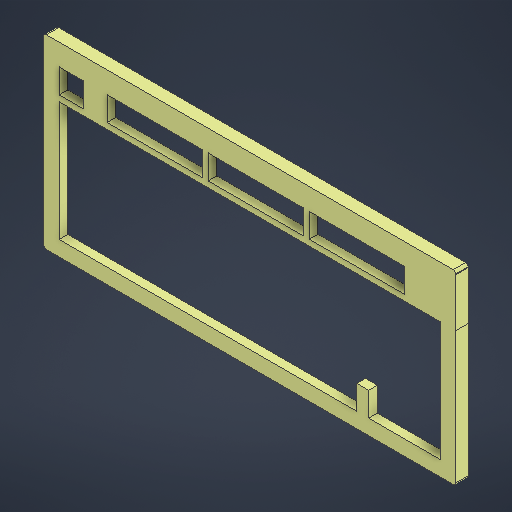
# Autodesk Inventor part: Keyboard_Case
Saved by Autodesk Inventor 2026.1 (Build 301233000, 233)
## iProperties
Created: 2025-11-09
Part Number: Keyboard_Case
Material: Generic
Document SubType Name: Modeling
Designer: avani
Density: 1 g/cm^3
Appearance: Default
Autodesk Inventor part; units mm, degrees
(part 1 of 5)
ref_plane "YZ Plane" through (0, 0, 0) normal (1, 0, 0) x (0, 1, 0)
ref_plane "XZ Plane" through (0, 0, 0) normal (0, 1, 0) x (-1, 0, 0)
sketch "Sketch1" plane through (0, 0, 0) normal (0, 0, 1) x (1, 0, 0)
  point P0 (0, 0)
sketch3d "3D 0"
sketch "Sketch2" plane through (0, 0, 0) normal (0, 0, 1) x (1, 0, 0)
  line L0 (303.652, 119.844) -> (303.808, 119.826) projected
  line L1 (303.808, 119.826) -> (303.962, 119.796) projected
  line L2 (303.962, 119.796) -> (304.115, 119.753) projected
  line L3 (304.115, 119.753) -> (304.261, 119.698) projected
  line L4 (304.261, 119.698) -> (304.403, 119.633) projected
  line L5 (304.403, 119.633) -> (304.541, 119.556) projected
  line L6 (304.672, 119.469) -> (304.794, 119.371) projected
  line L7 (304.541, 119.556) -> (304.672, 119.469) projected
  line L8 (304.794, 119.371) -> (304.91, 119.265) projected
  line L9 (304.91, 119.265) -> (305.016, 119.149) projected
  line L10 (305.016, 119.149) -> (305.114, 119.025) projected
  line L11 (305.114, 119.025) -> (305.201, 118.894) projected
  line L12 (305.201, 118.894) -> (305.278, 118.758) projected
  line L13 (305.278, 118.758) -> (305.343, 118.616) projected
  line L14 (305.343, 118.616) -> (305.398, 118.468) projected
  line L15 (305.398, 118.468) -> (305.441, 118.317) projected
  line L16 (305.441, 118.317) -> (305.471, 118.163) projected
  line L17 (305.471, 1.8741) -> (305.441, 1.7198) projected
  line L18 (305.398, 1.5696) -> (305.343, 1.4221) projected
  line L19 (305.343, 1.4221) -> (305.278, 1.2788) projected
  line L20 (305.278, 1.2788) -> (305.201, 1.1424) projected
  line L21 (305.201, 1.1424) -> (305.114, 1.0115) projected
  line L22 (305.441, 1.7198) -> (305.398, 1.5696) projected
  line L23 (305.114, 1.0115) -> (305.016, 0.8875) projected
  line L24 (305.016, 0.8875) -> (304.91, 0.7731) projected
  line L25 (304.794, 0.6656) -> (304.672, 0.5691) projected
  line L26 (304.672, 0.5691) -> (304.541, 0.4823) projected
  line L27 (304.541, 0.4823) -> (304.403, 0.4051) projected
  line L28 (304.91, 0.7731) -> (304.794, 0.6656) projected
  line L29 (304.403, 0.4051) -> (304.261, 0.339) projected
  line L30 (304.261, 0.339) -> (304.115, 0.2853) projected
  line L31 (304.115, 0.2853) -> (303.962, 0.2425) projected
  line L32 (303.962, 0.2425) -> (303.808, 0.2122) projected
  line L33 (303.808, 0.2122) -> (303.652, 0.1929) projected
  line L34 (303.652, 0.1929) -> (303.496, 0.1874) projected
  line L35 (305.471, 118.163) -> (305.489, 118.007) projected
  line L36 (305.489, 118.007) -> (305.496, 117.85) projected
  line L37 (305.496, 117.85) -> (305.496, 2.1869) projected
  line L38 (305.496, 2.1869) -> (305.489, 2.0299) projected
  line L39 (305.489, 2.0299) -> (305.471, 1.8741) projected
  line L40 (2.096, 119.849) -> (303.496, 119.849) projected
  line L41 (303.496, 0.1874) -> (2.096, 0.1874) projected
  line L42 (135.883, 116.926) -> (135.883, 103.125) projected
  line L43 (135.883, 103.125) -> (122.083, 103.125) projected
  line L44 (122.083, 116.926) -> (135.883, 116.926) projected
  line L45 (122.083, 103.125) -> (122.083, 116.926) projected
  line L46 (98.2694, 116.926) -> (112.07, 116.926) projected
  line L47 (112.07, 103.125) -> (98.2694, 103.125) projected
  line L48 (112.07, 116.926) -> (112.07, 103.125) projected
  line L49 (28.7266, 35.9625) -> (14.9269, 35.9625) projected
  line L50 (23.9641, 55.0125) -> (23.9641, 41.2129) projected
  line L51 (23.9641, 41.2129) -> (10.163, 41.2129) projected
  line L52 (10.163, 55.0125) -> (23.9641, 55.0125) projected
  line L53 (10.163, 41.2129) -> (10.163, 55.0125) projected
  line L54 (78.0881, 15.4423) -> (78.0881, 12.2136) projected
  line L55 (78.0881, 12.2136) -> (77.264, 12.2136) projected
  line L56 (77.264, 12.2136) -> (77.264, 9.6132) projected
  line L57 (77.264, 9.6132) -> (78.0881, 9.6132) projected
  line L58 (53.0271, 16.9127) -> (66.8267, 16.9127) projected
  line L59 (66.8267, 16.9127) -> (66.8267, 3.113) projected
  line L60 (53.0271, 3.113) -> (53.0271, 16.9127) projected
  line L61 (66.8267, 3.113) -> (53.0271, 3.113) projected
  line L62 (78.0881, 9.6132) -> (78.0881, 3.3431) projected
  line L63 (78.7329, 22.163) -> (64.9333, 22.163) projected
  line L64 (78.7329, 35.9625) -> (78.7329, 22.163) projected
  line L65 (64.9333, 35.9625) -> (78.7329, 35.9625) projected
  line L66 (69.2079, 41.2129) -> (55.4083, 41.2129) projected
  line L67 (69.2079, 55.0125) -> (69.2079, 41.2129) projected
  line L68 (55.4083, 55.0125) -> (69.2079, 55.0125) projected
  line L69 (55.4083, 41.2129) -> (55.4083, 55.0125) projected
  line L70 (50.1579, 55.0125) -> (50.1579, 41.2129) projected
  line L71 (50.1579, 41.2129) -> (36.3583, 41.2129) projected
  line L72 (36.3583, 55.0125) -> (50.1579, 55.0125) projected
  line L73 (36.3583, 41.2129) -> (36.3583, 55.0125) projected
  line L74 (84.6391, 15.4423) -> (78.0881, 15.4423) projected
  line L75 (78.0881, 3.3431) -> (79.8132, 3.3431) projected
  line L76 (84.6391, 3.3431) -> (84.6391, 7.8135) projected
  line L77 (82.9137, 3.3431) -> (84.6391, 3.3431) projected
  line L78 (82.9137, 2.1429) -> (82.9137, 3.3431) projected
  line L79 (79.8132, 2.1429) -> (82.9137, 2.1429) projected
  line L80 (79.8132, 3.3431) -> (79.8132, 2.1429) projected
  line L81 (21.5828, 60.2629) -> (7.7832, 60.2629) projected
  line L82 (7.7832, 74.0625) -> (21.5828, 74.0625) projected
  line L83 (7.7832, 60.2629) -> (7.7832, 74.0625) projected
  line L84 (21.5828, 74.0625) -> (21.5828, 60.2629) projected
  line L85 (31.5957, 60.2629) -> (31.5957, 74.0625) projected
  line L86 (35.8704, 79.3129) -> (22.0707, 79.3129) projected
  line L87 (45.3954, 60.2629) -> (31.5957, 60.2629) projected
  line L88 (31.5957, 74.0625) -> (45.3954, 74.0625) projected
  line L89 (45.3954, 74.0625) -> (45.3954, 60.2629) projected
  line L90 (0.0951, 2.1869) -> (0.0951, 117.85) projected
  line L91 (16.8203, 79.3129) -> (3.0193, 79.3129) projected
  line L92 (3.0193, 79.3129) -> (3.0193, 93.1125) projected
  line L93 (16.8203, 93.1125) -> (16.8203, 79.3129) projected
  line L94 (3.0193, 93.1125) -> (16.8203, 93.1125) projected
  line L95 (16.8203, 103.125) -> (3.0193, 103.125) projected
  line L96 (3.0193, 103.125) -> (3.0193, 116.926) projected
  line L97 (3.0193, 116.926) -> (16.8203, 116.926) projected
  line L98 (16.8203, 116.926) -> (16.8203, 103.125) projected
  line L99 (124.463, 12.2136) -> (84.6391, 12.2136) projected
  line L100 (84.6391, 12.2136) -> (84.6391, 15.4423) projected
  line L101 (84.6391, 7.8135) -> (124.463, 7.8135) projected
  line L102 (97.7829, 35.9625) -> (97.7829, 22.163) projected
  line L103 (103.033, 22.163) -> (103.033, 35.9625) projected
  line L104 (116.833, 22.163) -> (103.033, 22.163) projected
  line L105 (116.833, 35.9625) -> (116.833, 22.163) projected
  line L106 (103.033, 35.9625) -> (116.833, 35.9625) projected
  line L107 (97.7829, 22.163) -> (83.9833, 22.163) projected
  line L108 (83.9833, 22.163) -> (83.9833, 35.9625) projected
  line L109 (107.308, 41.2129) -> (93.5083, 41.2129) projected
  line L110 (83.9833, 35.9625) -> (97.7829, 35.9625) projected
  line L111 (93.5083, 55.0125) -> (107.308, 55.0125) projected
  line L112 (93.5083, 41.2129) -> (93.5083, 55.0125) projected
  line L113 (22.0707, 93.1125) -> (35.8704, 93.1125) projected
  line L114 (22.0707, 79.3129) -> (22.0707, 93.1125) projected
  line L115 (35.8704, 93.1125) -> (35.8704, 79.3129) projected
  line L116 (41.1208, 79.3129) -> (41.1208, 93.1125) projected
  line L117 (54.919, 79.3129) -> (41.1208, 79.3129) projected
  line L118 (54.919, 93.1125) -> (54.919, 79.3129) projected
  line L119 (74.4583, 41.2129) -> (74.4583, 55.0125) projected
  line L120 (83.4954, 60.2629) -> (69.6958, 60.2629) projected
  line L121 (69.6958, 60.2629) -> (69.6958, 74.0625) projected
  line L122 (83.4954, 74.0625) -> (83.4954, 60.2629) projected
  line L123 (74.4583, 55.0125) -> (88.2579, 55.0125) projected
  line L124 (88.2579, 55.0125) -> (88.2579, 41.2129) projected
  line L125 (88.2579, 41.2129) -> (74.4583, 41.2129) projected
  line L126 (50.6458, 74.0625) -> (64.4454, 74.0625) projected
  line L127 (64.4454, 74.0625) -> (64.4454, 60.2629) projected
  line L128 (64.4454, 60.2629) -> (50.6458, 60.2629) projected
  line L129 (50.6458, 60.2629) -> (50.6458, 74.0625) projected
  line L130 (73.9704, 79.3129) -> (60.1694, 79.3129) projected
  line L131 (79.2194, 79.3129) -> (79.2194, 93.1125) projected
  line L132 (73.9704, 93.1125) -> (73.9704, 79.3129) projected
  line L133 (60.1694, 93.1125) -> (73.9704, 93.1125) projected
  line L134 (60.1694, 79.3129) -> (60.1694, 93.1125) projected
  line L135 (69.6958, 74.0625) -> (83.4954, 74.0625) projected
  line L136 (107.794, 60.2629) -> (107.794, 74.0625) projected
  line L137 (102.545, 74.0625) -> (102.545, 60.2629) projected
  line L138 (102.545, 60.2629) -> (88.7444, 60.2629) projected
  line L139 (88.7444, 74.0625) -> (102.545, 74.0625) projected
  line L140 (88.7444, 60.2629) -> (88.7444, 74.0625) projected
  line L141 (54.919, 103.125) -> (41.1208, 103.125) projected
  line L142 (54.919, 116.926) -> (54.919, 103.125) projected
  line L143 (41.1208, 103.125) -> (41.1208, 116.926) projected
  line L144 (41.1208, 116.926) -> (54.919, 116.926) projected
  line L145 (41.1208, 93.1125) -> (54.919, 93.1125) projected
  line L146 (0.0951, 117.85) -> (0.102, 118.007) projected
  line L147 (0.102, 118.007) -> (0.1199, 118.163) projected
  line L148 (0.1199, 118.163) -> (0.1502, 118.317) projected
  line L149 (0.4768, 119.025) -> (0.5746, 119.149) projected
  line L150 (0.39, 118.894) -> (0.4768, 119.025) projected
  line L151 (0.3128, 118.758) -> (0.39, 118.894) projected
  line L152 (0.248, 118.616) -> (0.3128, 118.758) projected
  line L153 (0.1929, 118.468) -> (0.248, 118.616) projected
  line L154 (0.1502, 118.317) -> (0.1929, 118.468) projected
  line L155 (0.5746, 119.149) -> (0.6808, 119.265) projected
  line L156 (0.6808, 119.265) -> (0.7965, 119.371) projected
  line L157 (0.7965, 119.371) -> (0.9192, 119.469) projected
  line L158 (0.9192, 119.469) -> (1.0501, 119.556) projected
  line L159 (1.0501, 119.556) -> (1.1879, 119.633) projected
  line L160 (1.1879, 119.633) -> (1.3298, 119.698) projected
  line L161 (1.3298, 119.698) -> (1.4759, 119.753) projected
  line L162 (1.4759, 119.753) -> (1.6288, 119.796) projected
  line L163 (1.6288, 119.796) -> (1.7818, 119.826) projected
  line L164 (1.7818, 119.826) -> (1.9389, 119.844) projected
  line L165 (1.9389, 119.844) -> (2.096, 119.849) projected
  line L166 (107.308, 55.0125) -> (107.308, 41.2129) projected
  line L167 (112.558, 41.2129) -> (112.558, 55.0125) projected
  line L168 (126.358, 41.2129) -> (112.558, 41.2129) projected
  line L169 (126.358, 55.0125) -> (126.358, 41.2129) projected
  line L170 (112.558, 55.0125) -> (126.358, 55.0125) projected
  line L171 (121.595, 60.2629) -> (107.794, 60.2629) projected
  line L172 (107.794, 74.0625) -> (121.595, 74.0625) projected
  line L173 (121.595, 74.0625) -> (121.595, 60.2629) projected
  line L174 (93.0204, 79.3129) -> (79.2194, 79.3129) projected
  line L175 (93.0204, 93.1125) -> (93.0204, 79.3129) projected
  line L176 (79.2194, 93.1125) -> (93.0204, 93.1125) projected
  line L177 (93.0204, 103.125) -> (79.2194, 103.125) projected
  line L178 (98.2694, 103.125) -> (98.2694, 116.926) projected
  line L179 (145.896, 74.0625) -> (159.695, 74.0625) projected
  line L180 (159.695, 74.0625) -> (159.695, 60.2629) projected
  line L181 (145.896, 60.2629) -> (145.896, 74.0625) projected
  line L182 (140.645, 74.0625) -> (140.645, 60.2629) projected
  line L183 (140.645, 60.2629) -> (126.846, 60.2629) projected
  line L184 (126.846, 74.0625) -> (140.645, 74.0625) projected
  line L185 (126.846, 60.2629) -> (126.846, 74.0625) projected
  line L186 (112.07, 79.3129) -> (98.2694, 79.3129) projected
  line L187 (98.2694, 93.1125) -> (112.07, 93.1125) projected
  line L188 (98.2694, 79.3129) -> (98.2694, 93.1125) projected
  line L189 (131.12, 79.3129) -> (117.321, 79.3129) projected
  line L190 (112.07, 93.1125) -> (112.07, 79.3129) projected
  line L191 (117.321, 79.3129) -> (117.321, 93.1125) projected
  line L192 (131.12, 93.1125) -> (131.12, 79.3129) projected
  line L193 (117.321, 93.1125) -> (131.12, 93.1125) projected
  line L194 (79.2194, 116.926) -> (93.0204, 116.926) projected
  line L195 (93.0204, 116.926) -> (93.0204, 103.125) projected
  line L196 (79.2194, 103.125) -> (79.2194, 116.926) projected
  line L197 (73.9704, 103.125) -> (60.1694, 103.125) projected
  line L198 (73.9704, 116.926) -> (73.9704, 103.125) projected
  line L199 (60.1694, 103.125) -> (60.1694, 116.926) projected
  line L200 (60.1694, 116.926) -> (73.9704, 116.926) projected
  line L201 (141.133, 22.163) -> (141.133, 35.9625) projected
  line L202 (141.133, 35.9625) -> (154.933, 35.9625) projected
  line L203 (138.264, 7.8135) -> (178.088, 7.8135) projected
  line L204 (178.088, 12.2136) -> (138.264, 12.2136) projected
  line L205 (154.933, 35.9625) -> (154.933, 22.163) projected
  line L206 (178.088, 15.4423) -> (178.088, 12.2136) projected
  line L207 (160.183, 22.163) -> (160.183, 35.9625) projected
  line L208 (173.983, 22.163) -> (160.183, 22.163) projected
  line L209 (160.183, 35.9625) -> (173.983, 35.9625) projected
  line L210 (173.983, 35.9625) -> (173.983, 22.163) projected
  line L211 (184.638, 12.2136) -> (184.638, 15.4423) projected
  line L212 (184.638, 15.4423) -> (178.088, 15.4423) projected
  line L213 (193.033, 22.163) -> (179.233, 22.163) projected
  line L214 (179.233, 22.163) -> (179.233, 35.9625) projected
  line L215 (179.233, 35.9625) -> (193.033, 35.9625) projected
  line L216 (193.033, 35.9625) -> (193.033, 22.163) projected
  line L217 (178.088, 7.8135) -> (178.088, 3.3431) projected
  line L218 (178.088, 3.3431) -> (179.813, 3.3431) projected
  line L219 (179.813, 3.3431) -> (179.813, 2.1429) projected
  line L220 (179.813, 2.1429) -> (182.914, 2.1429) projected
  line L221 (182.914, 2.1429) -> (182.914, 3.3431) projected
  line L222 (185.463, 12.2136) -> (184.638, 12.2136) projected
  line L223 (185.463, 9.6132) -> (185.463, 12.2136) projected
  line L224 (184.638, 9.6132) -> (185.463, 9.6132) projected
  line L225 (184.638, 3.3431) -> (184.638, 9.6132) projected
  line L226 (182.914, 3.3431) -> (184.638, 3.3431) projected
  line L227 (195.902, 16.9127) -> (209.702, 16.9127) projected
  line L228 (209.702, 16.9127) -> (209.702, 3.113) projected
  line L229 (209.702, 3.113) -> (195.902, 3.113) projected
  line L230 (195.902, 3.113) -> (195.902, 16.9127) projected
  line L231 (124.463, 16.9127) -> (124.463, 12.2136) projected
  line L232 (124.463, 7.8135) -> (124.463, 3.113) projected
  line L233 (124.463, 3.113) -> (138.264, 3.113) projected
  line L234 (138.264, 12.2136) -> (138.264, 16.9127) projected
  line L235 (138.264, 16.9127) -> (124.463, 16.9127) projected
  line L236 (122.083, 35.9625) -> (135.883, 35.9625) projected
  line L237 (135.883, 22.163) -> (122.083, 22.163) projected
  line L238 (122.083, 22.163) -> (122.083, 35.9625) projected
  line L239 (135.883, 35.9625) -> (135.883, 22.163) projected
  line L240 (138.264, 3.113) -> (138.264, 7.8135) projected
  line L241 (154.933, 22.163) -> (141.133, 22.163) projected
  line L242 (202.558, 41.2129) -> (188.758, 41.2129) projected
  line L243 (188.758, 41.2129) -> (188.758, 55.0125) projected
  line L244 (188.758, 55.0125) -> (202.558, 55.0125) projected
  line L245 (202.558, 55.0125) -> (202.558, 41.2129) projected
  line L246 (221.608, 55.0125) -> (221.608, 41.2129) projected
  line L247 (226.858, 41.2129) -> (226.858, 55.0125) projected
  line L248 (240.658, 41.2129) -> (226.858, 41.2129) projected
  line L249 (240.658, 55.0125) -> (240.658, 41.2129) projected
  line L250 (257.813, 55.0125) -> (257.813, 50.3135) projected
  line L251 (257.813, 50.3135) -> (256.089, 50.3135) projected
  line L252 (256.089, 50.3135) -> (256.089, 53.5421) projected
  line L253 (256.089, 53.5421) -> (249.538, 53.5421) projected
  line L254 (248.714, 47.7132) -> (249.538, 47.7132) projected
  line L255 (249.538, 50.3135) -> (248.714, 50.3135) projected
  line L256 (248.714, 50.3135) -> (248.714, 47.7132) projected
  line L257 (249.538, 53.5421) -> (249.538, 50.3135) projected
  line L258 (257.813, 45.9133) -> (257.813, 41.2129) projected
  line L259 (256.089, 45.9133) -> (257.813, 45.9133) projected
  line L260 (257.813, 41.2129) -> (271.614, 41.2129) projected
  line L261 (256.089, 41.4433) -> (256.089, 45.9133) projected
  line L262 (271.614, 45.9133) -> (273.338, 45.9133) projected
  line L263 (273.338, 45.9133) -> (273.338, 41.4433) projected
  line L264 (273.338, 41.4433) -> (275.063, 41.4433) projected
  line L265 (271.614, 41.2129) -> (271.614, 45.9133) projected
  line L266 (273.338, 50.3135) -> (271.614, 50.3135) projected
  line L267 (271.614, 50.3135) -> (271.614, 55.0125) projected
  line L268 (273.338, 53.5421) -> (273.338, 50.3135) projected
  line L269 (278.758, 60.2629) -> (264.958, 60.2629) projected
  line L270 (271.614, 55.0125) -> (257.813, 55.0125) projected
  line L271 (278.758, 74.0625) -> (278.758, 60.2629) projected
  line L272 (264.958, 74.0625) -> (278.758, 74.0625) projected
  line L273 (264.958, 60.2629) -> (264.958, 74.0625) projected
  line L274 (260.196, 79.3129) -> (273.995, 79.3129) projected
  line L275 (150.17, 79.3129) -> (136.371, 79.3129) projected
  line L276 (169.22, 79.3129) -> (155.421, 79.3129) projected
  line L277 (136.371, 93.1125) -> (150.17, 93.1125) projected
  line L278 (136.371, 79.3129) -> (136.371, 93.1125) projected
  line L279 (150.17, 93.1125) -> (150.17, 79.3129) projected
  line L280 (155.421, 79.3129) -> (155.421, 93.1125) projected
  line L281 (169.22, 93.1125) -> (169.22, 79.3129) projected
  line L282 (155.421, 93.1125) -> (169.22, 93.1125) projected
  line L283 (173.983, 103.125) -> (160.183, 103.125) projected
  line L284 (154.933, 103.125) -> (141.133, 103.125) projected
  line L285 (141.133, 103.125) -> (141.133, 116.926) projected
  line L286 (141.133, 116.926) -> (154.933, 116.926) projected
  line L287 (154.933, 116.926) -> (154.933, 103.125) projected
  line L288 (160.183, 103.125) -> (160.183, 116.926) projected
  line L289 (160.183, 116.926) -> (173.983, 116.926) projected
  line L290 (173.983, 116.926) -> (173.983, 103.125) projected
  line L291 (178.745, 74.0625) -> (178.745, 60.2629) projected
  line L292 (178.745, 60.2629) -> (164.946, 60.2629) projected
  line L293 (164.946, 60.2629) -> (164.946, 74.0625) projected
  line L294 (164.946, 74.0625) -> (178.745, 74.0625) projected
  line L295 (197.795, 60.2629) -> (183.996, 60.2629) projected
  line L296 (197.795, 74.0625) -> (197.795, 60.2629) projected
  line L297 (183.996, 60.2629) -> (183.996, 74.0625) projected
  line L298 (183.996, 74.0625) -> (197.795, 74.0625) projected
  line L299 (183.508, 55.0125) -> (183.508, 41.2129) projected
  line L300 (183.508, 41.2129) -> (169.708, 41.2129) projected
  line L301 (169.708, 41.2129) -> (169.708, 55.0125) projected
  line L302 (169.708, 55.0125) -> (183.508, 55.0125) projected
  line L303 (188.27, 79.3129) -> (174.471, 79.3129) projected
  line L304 (207.32, 79.3129) -> (193.521, 79.3129) projected
  line L305 (174.471, 93.1125) -> (188.27, 93.1125) projected
  line L306 (174.471, 79.3129) -> (174.471, 93.1125) projected
  line L307 (188.27, 93.1125) -> (188.27, 79.3129) projected
  line L308 (193.521, 79.3129) -> (193.521, 93.1125) projected
  line L309 (207.32, 93.1125) -> (207.32, 79.3129) projected
  line L310 (193.521, 93.1125) -> (207.32, 93.1125) projected
  line L311 (216.845, 74.0625) -> (216.845, 60.2629) projected
  line L312 (216.845, 60.2629) -> (203.046, 60.2629) projected
  line L313 (203.046, 60.2629) -> (203.046, 74.0625) projected
  line L314 (203.046, 74.0625) -> (216.845, 74.0625) projected
  line L315 (216.845, 103.125) -> (203.046, 103.125) projected
  line L316 (193.033, 103.125) -> (179.233, 103.125) projected
  line L317 (179.233, 103.125) -> (179.233, 116.926) projected
  line L318 (179.233, 116.926) -> (193.033, 116.926) projected
  line L319 (193.033, 116.926) -> (193.033, 103.125) projected
  line L320 (203.046, 103.125) -> (203.046, 116.926) projected
  line L321 (216.845, 116.926) -> (216.845, 103.125) projected
  line L322 (203.046, 116.926) -> (216.845, 116.926) projected
  line L323 (235.895, 60.2629) -> (222.096, 60.2629) projected
  line L324 (222.096, 60.2629) -> (222.096, 74.0625) projected
  line L325 (222.096, 74.0625) -> (235.895, 74.0625) projected
  line L326 (235.895, 74.0625) -> (235.895, 60.2629) projected
  line L327 (226.858, 55.0125) -> (240.658, 55.0125) projected
  line L328 (198.283, 35.9625) -> (212.083, 35.9625) projected
  line L329 (212.083, 35.9625) -> (212.083, 22.163) projected
  line L330 (212.083, 22.163) -> (198.283, 22.163) projected
  line L331 (207.808, 55.0125) -> (221.608, 55.0125) projected
  line L332 (207.808, 41.2129) -> (207.808, 55.0125) projected
  line L333 (217.333, 35.9625) -> (231.133, 35.9625) projected
  line L334 (231.133, 35.9625) -> (231.133, 22.163) projected
  line L335 (231.133, 22.163) -> (217.333, 22.163) projected
  line L336 (221.608, 41.2129) -> (207.808, 41.2129) projected
  line L337 (198.283, 22.163) -> (198.283, 35.9625) projected
  line L338 (217.333, 22.163) -> (217.333, 35.9625) projected
  line L339 (226.37, 79.3129) -> (212.571, 79.3129) projected
  line L340 (245.42, 79.3129) -> (231.621, 79.3129) projected
  line L341 (212.571, 93.1125) -> (226.37, 93.1125) projected
  line L342 (212.571, 79.3129) -> (212.571, 93.1125) projected
  line L343 (226.37, 93.1125) -> (226.37, 79.3129) projected
  line L344 (231.621, 79.3129) -> (231.621, 93.1125) projected
  line L345 (245.42, 93.1125) -> (245.42, 79.3129) projected
  line L346 (231.621, 93.1125) -> (245.42, 93.1125) projected
  line L347 (235.895, 103.125) -> (222.096, 103.125) projected
  line L348 (254.945, 103.125) -> (241.146, 103.125) projected
  line L349 (241.146, 116.926) -> (254.945, 116.926) projected
  line L350 (241.146, 103.125) -> (241.146, 116.926) projected
  line L351 (222.096, 103.125) -> (222.096, 116.926) projected
  line L352 (222.096, 116.926) -> (235.895, 116.926) projected
  line L353 (235.895, 116.926) -> (235.895, 103.125) projected
  line L354 (241.146, 74.0625) -> (254.945, 74.0625) projected
  line L355 (254.945, 74.0625) -> (254.945, 60.2629) projected
  line L356 (254.945, 60.2629) -> (241.146, 60.2629) projected
  line L357 (241.146, 60.2629) -> (241.146, 74.0625) projected
  line L358 (251.92, 85.8132) -> (251.92, 79.5433) projected
  line L359 (251.92, 79.5433) -> (253.646, 79.5433) projected
  line L360 (256.745, 78.3428) -> (256.745, 79.5433) projected
  line L361 (253.646, 79.5433) -> (253.646, 78.3428) projected
  line L362 (253.646, 78.3428) -> (256.745, 78.3428) projected
  line L363 (256.745, 79.5433) -> (258.47, 79.5433) projected
  line L364 (260.196, 84.0133) -> (260.196, 79.3129) projected
  line L365 (258.47, 84.0133) -> (260.196, 84.0133) projected
  line L366 (258.47, 79.5433) -> (258.47, 84.0133) projected
  line L367 (260.196, 93.1125) -> (260.196, 88.4135) projected
  line L368 (260.196, 88.4135) -> (258.47, 88.4135) projected
  line L369 (251.095, 85.8132) -> (251.92, 85.8132) projected
  line L370 (251.095, 88.4135) -> (251.095, 85.8132) projected
  line L371 (251.92, 88.4135) -> (251.095, 88.4135) projected
  line L372 (251.92, 91.6421) -> (251.92, 88.4135) projected
  line L373 (258.47, 91.6421) -> (251.92, 91.6421) projected
  line L374 (258.47, 88.4135) -> (258.47, 91.6421) projected
  line L375 (273.995, 93.1125) -> (260.196, 93.1125) projected
  line L376 (273.995, 103.125) -> (260.196, 103.125) projected
  line L377 (273.995, 116.926) -> (273.995, 103.125) projected
  line L378 (260.196, 116.926) -> (273.995, 116.926) projected
  line L379 (260.196, 103.125) -> (260.196, 116.926) projected
  line L380 (254.945, 116.926) -> (254.945, 103.125) projected
  line L381 (249.538, 47.7132) -> (249.538, 41.4433) projected
  line L382 (249.538, 41.4433) -> (251.263, 41.4433) projected
  line L383 (251.263, 41.4433) -> (251.263, 40.2428) projected
  line L384 (251.263, 40.2428) -> (254.362, 40.2428) projected
  line L385 (254.362, 40.2428) -> (254.362, 41.4433) projected
  line L386 (254.362, 41.4433) -> (256.089, 41.4433) projected
  line L387 (164.458, 41.2129) -> (150.658, 41.2129) projected
  line L388 (164.458, 55.0125) -> (164.458, 41.2129) projected
  line L389 (150.658, 55.0125) -> (164.458, 55.0125) projected
  line L390 (150.658, 41.2129) -> (150.658, 55.0125) projected
  line L391 (159.695, 60.2629) -> (145.896, 60.2629) projected
  line L392 (145.408, 55.0125) -> (145.408, 41.2129) projected
  line L393 (145.408, 41.2129) -> (131.608, 41.2129) projected
  line L394 (131.608, 55.0125) -> (145.408, 55.0125) projected
  line L395 (131.608, 41.2129) -> (131.608, 55.0125) projected
  line L396 (0.7965, 0.6656) -> (0.6808, 0.7731) projected
  line L397 (0.6808, 0.7731) -> (0.5746, 0.8875) projected
  line L398 (0.5746, 0.8875) -> (0.4768, 1.0115) projected
  line L399 (0.4768, 1.0115) -> (0.39, 1.1424) projected
  line L400 (0.39, 1.1424) -> (0.3128, 1.2788) projected
  line L401 (0.3128, 1.2788) -> (0.248, 1.4221) projected
  line L402 (14.9269, 35.9625) -> (14.9269, 31.2636) projected
  line L403 (14.9269, 31.2636) -> (13.2016, 31.2636) projected
  line L404 (13.2016, 31.2636) -> (13.2016, 34.4923) projected
  line L405 (13.2016, 34.4923) -> (6.6518, 34.4923) projected
  line L406 (6.6518, 34.4923) -> (6.6518, 31.2636) projected
  line L407 (6.6518, 31.2636) -> (5.8263, 31.2636) projected
  line L408 (5.8263, 31.2636) -> (5.8263, 28.6632) projected
  line L409 (5.8263, 28.6632) -> (6.6518, 28.6632) projected
  line L410 (30.4519, 26.8635) -> (30.4519, 22.3931) projected
  line L411 (30.4519, 22.3931) -> (32.1758, 22.3931) projected
  line L412 (32.1758, 22.3931) -> (32.1758, 21.1928) projected
  line L413 (32.1758, 21.1928) -> (35.2764, 21.1928) projected
  line L414 (35.2764, 21.1928) -> (35.2764, 22.3931) projected
  line L415 (35.2764, 22.3931) -> (37.0018, 22.3931) projected
  line L416 (37.0018, 22.3931) -> (37.0018, 28.6632) projected
  line L417 (37.0018, 28.6632) -> (37.8273, 28.6632) projected
  line L418 (37.8273, 28.6632) -> (37.8273, 31.2636) projected
  line L419 (37.8273, 31.2636) -> (37.0018, 31.2636) projected
  line L420 (37.0018, 31.2636) -> (37.0018, 34.4923) projected
  line L421 (37.0018, 34.4923) -> (30.4519, 34.4923) projected
  line L422 (30.4519, 31.2636) -> (28.7266, 31.2636) projected
  line L423 (28.7266, 31.2636) -> (28.7266, 35.9625) projected
  line L424 (30.4519, 34.4923) -> (30.4519, 31.2636) projected
  line L425 (13.2016, 26.8635) -> (14.9269, 26.8635) projected
  line L426 (13.2016, 22.3931) -> (13.2016, 26.8635) projected
  line L427 (6.6518, 28.6632) -> (6.6518, 22.3931) projected
  line L428 (6.6518, 22.3931) -> (8.3771, 22.3931) projected
  line L429 (29.213, 16.9127) -> (43.0142, 16.9127) projected
  line L430 (43.0142, 16.9127) -> (43.0142, 3.113) projected
  line L431 (43.0142, 3.113) -> (29.213, 3.113) projected
  line L432 (29.213, 3.113) -> (29.213, 16.9127) projected
  line L433 (14.9269, 26.8635) -> (14.9269, 22.163) projected
  line L434 (14.9269, 22.163) -> (28.7266, 22.163) projected
  line L435 (28.7266, 22.163) -> (28.7266, 26.8635) projected
  line L436 (28.7266, 26.8635) -> (30.4519, 26.8635) projected
  line L437 (8.3771, 22.3931) -> (8.3771, 21.1928) projected
  line L438 (11.4763, 21.1928) -> (11.4763, 22.3931) projected
  line L439 (8.3771, 21.1928) -> (11.4763, 21.1928) projected
  line L440 (5.4019, 16.9127) -> (19.2016, 16.9127) projected
  line L441 (5.4019, 3.113) -> (5.4019, 16.9127) projected
  line L442 (19.2016, 3.113) -> (5.4019, 3.113) projected
  line L443 (19.2016, 16.9127) -> (19.2016, 3.113) projected
  line L444 (11.4763, 22.3931) -> (13.2016, 22.3931) projected
  line L445 (0.248, 1.4221) -> (0.1929, 1.5696) projected
  line L446 (0.1929, 1.5696) -> (0.1502, 1.7198) projected
  line L447 (0.1502, 1.7198) -> (0.1199, 1.8741) projected
  line L448 (0.1199, 1.8741) -> (0.102, 2.0299) projected
  line L449 (0.102, 2.0299) -> (0.0951, 2.1869) projected
  line L450 (2.096, 0.1874) -> (1.9389, 0.1929) projected
  line L451 (1.9389, 0.1929) -> (1.7818, 0.2122) projected
  line L452 (1.7818, 0.2122) -> (1.6288, 0.2425) projected
  line L453 (0.9192, 0.5691) -> (0.7965, 0.6656) projected
  line L454 (1.0501, 0.4823) -> (0.9192, 0.5691) projected
  line L455 (1.3298, 0.339) -> (1.1879, 0.4051) projected
  line L456 (1.4759, 0.2853) -> (1.3298, 0.339) projected
  line L457 (1.6288, 0.2425) -> (1.4759, 0.2853) projected
  line L458 (1.1879, 0.4051) -> (1.0501, 0.4823) projected
  line L459 (64.9333, 22.163) -> (64.9333, 35.9625) projected
  line L460 (59.6829, 35.9625) -> (59.6829, 22.163) projected
  line L461 (59.6829, 22.163) -> (45.8833, 22.163) projected
  line L462 (45.8833, 22.163) -> (45.8833, 35.9625) projected
  line L463 (45.8833, 35.9625) -> (59.6829, 35.9625) projected
  line L464 (288.771, 35.9625) -> (302.57, 35.9625) projected
  line L465 (302.57, 35.9625) -> (302.57, 22.163) projected
  line L466 (288.771, 22.163) -> (288.771, 35.9625) projected
  line L467 (283.52, 22.163) -> (269.721, 22.163) projected
  line L468 (269.721, 35.9625) -> (283.52, 35.9625) projected
  line L469 (269.721, 22.163) -> (269.721, 35.9625) projected
  line L470 (283.52, 35.9625) -> (283.52, 22.163) projected
  line L471 (269.721, 16.9127) -> (283.52, 16.9127) projected
  line L472 (283.52, 16.9127) -> (283.52, 3.113) projected
  line L473 (283.52, 3.113) -> (269.721, 3.113) projected
  line L474 (269.721, 3.113) -> (269.721, 16.9127) projected
  line L475 (302.57, 22.163) -> (288.771, 22.163) projected
  line L476 (288.771, 16.9127) -> (302.57, 16.9127) projected
  line L477 (288.771, 3.113) -> (288.771, 16.9127) projected
  line L478 (302.57, 16.9127) -> (302.57, 3.113) projected
  line L479 (302.57, 3.113) -> (288.771, 3.113) projected
  line L480 (302.57, 41.2129) -> (288.771, 41.2129) projected
  line L481 (279.888, 47.7132) -> (280.713, 47.7132) projected
  line L482 (280.713, 50.3135) -> (279.888, 50.3135) projected
  line L483 (280.713, 47.7132) -> (280.713, 50.3135) projected
  line L484 (279.888, 50.3135) -> (279.888, 53.5421) projected
  line L485 (288.771, 41.2129) -> (288.771, 55.0125) projected
  line L486 (302.57, 55.0125) -> (302.57, 41.2129) projected
  line L487 (219.713, 16.9127) -> (233.514, 16.9127) projected
  line L488 (233.514, 16.9127) -> (233.514, 3.113) projected
  line L489 (233.514, 3.113) -> (219.713, 3.113) projected
  line L490 (219.713, 3.113) -> (219.713, 16.9127) projected
  line L491 (250.671, 16.9127) -> (264.47, 16.9127) projected
  line L492 (264.47, 16.9127) -> (264.47, 3.113) projected
  line L493 (264.47, 3.113) -> (250.671, 3.113) projected
  line L494 (250.671, 3.113) -> (250.671, 16.9127) projected
  line L495 (288.771, 55.0125) -> (302.57, 55.0125) projected
  line L496 (302.57, 60.2629) -> (288.771, 60.2629) projected
  line L497 (288.771, 60.2629) -> (288.771, 74.0625) projected
  line L498 (302.57, 74.0625) -> (302.57, 60.2629) projected
  line L499 (288.771, 74.0625) -> (302.57, 74.0625) projected
  line L500 (277.446, 78.3428) -> (280.545, 78.3428) projected
  line L501 (277.446, 79.5433) -> (277.446, 78.3428) projected
  line L502 (275.721, 79.5433) -> (277.446, 79.5433) projected
  line L503 (273.995, 79.3129) -> (273.995, 84.0133) projected
  line L504 (273.995, 84.0133) -> (275.721, 84.0133) projected
  line L505 (275.721, 84.0133) -> (275.721, 79.5433) projected
  line L506 (282.271, 88.4135) -> (282.271, 91.6421) projected
  line L507 (275.721, 88.4135) -> (273.995, 88.4135) projected
  line L508 (275.721, 91.6421) -> (275.721, 88.4135) projected
  line L509 (273.995, 88.4135) -> (273.995, 93.1125) projected
  line L510 (282.271, 91.6421) -> (275.721, 91.6421) projected
  line L511 (280.545, 79.5433) -> (282.271, 79.5433) projected
  line L512 (282.271, 79.5433) -> (282.271, 85.8132) projected
  line L513 (282.271, 85.8132) -> (283.096, 85.8132) projected
  line L514 (283.096, 88.4135) -> (282.271, 88.4135) projected
  line L515 (283.096, 85.8132) -> (283.096, 88.4135) projected
  line L516 (280.545, 78.3428) -> (280.545, 79.5433) projected
  line L517 (243.527, 35.9625) -> (257.327, 35.9625) projected
  line L518 (257.327, 35.9625) -> (257.327, 22.163) projected
  line L519 (257.327, 22.163) -> (243.527, 22.163) projected
  line L520 (243.527, 22.163) -> (243.527, 35.9625) projected
  line L521 (279.888, 41.4433) -> (279.888, 47.7132) projected
  line L522 (278.164, 41.4433) -> (279.888, 41.4433) projected
  line L523 (279.888, 53.5421) -> (273.338, 53.5421) projected
  line L524 (275.063, 41.4433) -> (275.063, 40.2428) projected
  line L525 (275.063, 40.2428) -> (278.164, 40.2428) projected
  line L526 (278.164, 40.2428) -> (278.164, 41.4433) projected
  line L527 (303.496, 119.849) -> (303.652, 119.844) projected
  line L528 (288.771, 79.3129) -> (288.771, 93.1125) projected
  line L529 (288.771, 93.1125) -> (302.57, 93.1125) projected
  line L530 (302.57, 93.1125) -> (302.57, 79.3129) projected
  line L531 (302.57, 79.3129) -> (288.771, 79.3129) projected
  point P0 (0, 0)
  point P1 (0, 0)
ref_plane "Work Plane1" through (0, 0, 1.5) normal (0, 0, 1) x (1, 0, 0)
sketch "Sketch3" plane through (0, 0, 1.5) normal (0, 0, 1) x (1, 0, 0)
  line L0 (258.47, 91.6421) -> (258.47, 88.4135) projected
  line L1 (251.92, 91.6421) -> (258.47, 91.6421) projected
  line L2 (251.095, 88.4135) -> (251.92, 88.4135) projected
  line L3 (254.945, 103.125) -> (241.146, 103.125) projected
  line L4 (254.945, 103.125) -> (241.146, 103.125) projected
  line L5 (254.945, 103.125) -> (241.146, 103.125) projected
  line L6 (254.945, 103.125) -> (241.146, 103.125) projected
  line L7 (235.895, 116.926) -> (235.895, 103.125) projected
  line L8 (235.895, 116.926) -> (235.895, 103.125) projected
  line L9 (241.146, 103.125) -> (241.146, 116.926) projected
  line L10 (241.146, 103.125) -> (241.146, 116.926) projected
  line L11 (241.146, 103.125) -> (241.146, 116.926) projected
  line L12 (241.146, 103.125) -> (241.146, 116.926) projected
  line L13 (241.146, 116.926) -> (254.945, 116.926) projected
  line L14 (241.146, 116.926) -> (254.945, 116.926) projected
  line L15 (241.146, 116.926) -> (254.945, 116.926) projected
  line L16 (241.146, 116.926) -> (254.945, 116.926) projected
  line L17 (254.945, 116.926) -> (254.945, 103.125) projected
  line L18 (254.945, 116.926) -> (254.945, 103.125) projected
  line L19 (254.945, 116.926) -> (254.945, 103.125) projected
  line L20 (254.945, 116.926) -> (254.945, 103.125) projected
  line L21 (273.995, 103.125) -> (260.196, 103.125) projected
  line L22 (273.995, 103.125) -> (260.196, 103.125) projected
  line L23 (260.196, 103.125) -> (260.196, 116.926) projected
  line L24 (260.196, 103.125) -> (260.196, 116.926) projected
  line L25 (260.196, 116.926) -> (273.995, 116.926) projected
  line L26 (260.196, 116.926) -> (273.995, 116.926) projected
  line L27 (273.995, 116.926) -> (273.995, 103.125) projected
  line L28 (273.995, 116.926) -> (273.995, 103.125) projected
  line L29 (260.196, 103.125) -> (260.196, 116.926) projected
  line L30 (260.196, 103.125) -> (260.196, 116.926) projected
  line L31 (273.995, 103.125) -> (260.196, 103.125) projected
  line L32 (273.995, 103.125) -> (260.196, 103.125) projected
  line L33 (273.995, 116.926) -> (273.995, 103.125) projected
  line L34 (273.995, 116.926) -> (273.995, 103.125) projected
  line L35 (260.196, 116.926) -> (273.995, 116.926) projected
  line L36 (260.196, 116.926) -> (273.995, 116.926) projected
  line L37 (260.196, 88.4135) -> (260.196, 93.1125) projected
  line L38 (260.196, 88.4135) -> (260.196, 93.1125) projected
  line L39 (260.196, 93.1125) -> (273.995, 93.1125) projected
  line L40 (260.196, 93.1125) -> (273.995, 93.1125) projected
  line L41 (273.995, 88.4135) -> (275.721, 88.4135) projected
  line L42 (273.995, 88.4135) -> (275.721, 88.4135) projected
  line L43 (273.995, 93.1125) -> (273.995, 88.4135) projected
  line L44 (273.995, 93.1125) -> (273.995, 88.4135) projected
  line L45 (275.721, 88.4135) -> (275.721, 91.6421) projected
  line L46 (275.721, 88.4135) -> (275.721, 91.6421) projected
  line L47 (275.721, 91.6421) -> (282.271, 91.6421) projected
  line L48 (275.721, 91.6421) -> (282.271, 91.6421) projected
  line L49 (305.496, 117.85) -> (305.489, 118.007) projected
  line L50 (305.496, 117.85) -> (305.489, 118.007) projected
  line L51 (305.489, 118.007) -> (305.471, 118.163) projected
  line L52 (305.489, 118.007) -> (305.471, 118.163) projected
  line L53 (305.441, 118.317) -> (305.398, 118.468) projected
  line L54 (305.441, 118.317) -> (305.398, 118.468) projected
  line L55 (305.441, 118.317) -> (305.398, 118.468) projected
  line L56 (305.441, 118.317) -> (305.398, 118.468) projected
  line L57 (305.471, 118.163) -> (305.441, 118.317) projected
  line L58 (305.471, 118.163) -> (305.441, 118.317) projected
  line L59 (305.471, 118.163) -> (305.441, 118.317) projected
  line L60 (305.489, 118.007) -> (305.471, 118.163) projected
  line L61 (305.489, 118.007) -> (305.471, 118.163) projected
  line L62 (305.496, 117.85) -> (305.489, 118.007) projected
  line L63 (305.496, 117.85) -> (305.489, 118.007) projected
  line L64 (305.471, 118.163) -> (305.441, 118.317) projected
  line L65 (305.398, 118.468) -> (305.343, 118.616) projected
  line L66 (305.398, 118.468) -> (305.343, 118.616) projected
  line L67 (305.343, 118.616) -> (305.278, 118.758) projected
  line L68 (305.343, 118.616) -> (305.278, 118.758) projected
  line L69 (305.343, 118.616) -> (305.278, 118.758) projected
  line L70 (305.343, 118.616) -> (305.278, 118.758) projected
  line L71 (305.278, 118.758) -> (305.201, 118.894) projected
  line L72 (305.278, 118.758) -> (305.201, 118.894) projected
  line L73 (305.278, 118.758) -> (305.201, 118.894) projected
  line L74 (305.278, 118.758) -> (305.201, 118.894) projected
  line L75 (305.201, 118.894) -> (305.114, 119.025) projected
  line L76 (305.201, 118.894) -> (305.114, 119.025) projected
  line L77 (305.201, 118.894) -> (305.114, 119.025) projected
  line L78 (305.114, 119.025) -> (305.016, 119.149) projected
  line L79 (305.114, 119.025) -> (305.016, 119.149) projected
  line L80 (305.114, 119.025) -> (305.016, 119.149) projected
  line L81 (305.114, 119.025) -> (305.016, 119.149) projected
  line L82 (305.016, 119.149) -> (304.91, 119.265) projected
  line L83 (305.016, 119.149) -> (304.91, 119.265) projected
  line L84 (305.016, 119.149) -> (304.91, 119.265) projected
  line L85 (305.016, 119.149) -> (304.91, 119.265) projected
  line L86 (305.398, 118.468) -> (305.343, 118.616) projected
  line L87 (305.398, 118.468) -> (305.343, 118.616) projected
  line L88 (304.261, 119.698) -> (304.115, 119.753) projected
  line L89 (304.261, 119.698) -> (304.115, 119.753) projected
  line L90 (304.261, 119.698) -> (304.115, 119.753) projected
  line L91 (304.261, 119.698) -> (304.115, 119.753) projected
  line L92 (304.115, 119.753) -> (303.962, 119.796) projected
  line L93 (304.115, 119.753) -> (303.962, 119.796) projected
  line L94 (304.115, 119.753) -> (303.962, 119.796) projected
  line L95 (304.115, 119.753) -> (303.962, 119.796) projected
  line L96 (303.962, 119.796) -> (303.808, 119.826) projected
  line L97 (303.962, 119.796) -> (303.808, 119.826) projected
  line L98 (303.962, 119.796) -> (303.808, 119.826) projected
  line L99 (303.962, 119.796) -> (303.808, 119.826) projected
  line L100 (303.808, 119.826) -> (303.652, 119.844) projected
  line L101 (303.808, 119.826) -> (303.652, 119.844) projected
  line L102 (303.808, 119.826) -> (303.652, 119.844) projected
  line L103 (303.652, 119.844) -> (303.496, 119.849) projected
  line L104 (303.652, 119.844) -> (303.496, 119.849) projected
  line L105 (303.652, 119.844) -> (303.496, 119.849) projected
  line L106 (305.201, 118.894) -> (305.114, 119.025) projected
  line L107 (304.91, 119.265) -> (304.794, 119.371) projected
  line L108 (304.91, 119.265) -> (304.794, 119.371) projected
  line L109 (304.794, 119.371) -> (304.672, 119.469) projected
  line L110 (304.794, 119.371) -> (304.672, 119.469) projected
  line L111 (304.403, 119.633) -> (304.261, 119.698) projected
  line L112 (304.403, 119.633) -> (304.261, 119.698) projected
  line L113 (304.541, 119.556) -> (304.403, 119.633) projected
  line L114 (304.541, 119.556) -> (304.403, 119.633) projected
  line L115 (304.541, 119.556) -> (304.403, 119.633) projected
  line L116 (304.541, 119.556) -> (304.403, 119.633) projected
  line L117 (304.672, 119.469) -> (304.541, 119.556) projected
  line L118 (304.672, 119.469) -> (304.541, 119.556) projected
  line L119 (304.672, 119.469) -> (304.541, 119.556) projected
  line L120 (304.672, 119.469) -> (304.541, 119.556) projected
  line L121 (304.794, 119.371) -> (304.672, 119.469) projected
  line L122 (304.794, 119.371) -> (304.672, 119.469) projected
  line L123 (304.91, 119.265) -> (304.794, 119.371) projected
  line L124 (304.91, 119.265) -> (304.794, 119.371) projected
  line L125 (304.403, 119.633) -> (304.261, 119.698) projected
  line L126 (304.403, 119.633) -> (304.261, 119.698) projected
  line L127 (282.271, 79.5433) -> (280.545, 79.5433) projected
  line L128 (277.446, 78.3428) -> (277.446, 79.5433) projected
  line L129 (277.446, 78.3428) -> (277.446, 79.5433) projected
  line L130 (277.446, 79.5433) -> (275.721, 79.5433) projected
  line L131 (280.545, 78.3428) -> (277.446, 78.3428) projected
  line L132 (280.545, 78.3428) -> (277.446, 78.3428) projected
  line L133 (280.545, 79.5433) -> (280.545, 78.3428) projected
  line L134 (280.545, 79.5433) -> (280.545, 78.3428) projected
  line L135 (282.271, 79.5433) -> (280.545, 79.5433) projected
  line L136 (277.446, 79.5433) -> (275.721, 79.5433) projected
  line L137 (288.771, 79.3129) -> (288.771, 93.1125) projected
  line L138 (288.771, 79.3129) -> (288.771, 93.1125) projected
  line L139 (288.771, 93.1125) -> (302.57, 93.1125) projected
  line L140 (288.771, 93.1125) -> (302.57, 93.1125) projected
  line L141 (302.57, 93.1125) -> (302.57, 79.3129) projected
  line L142 (302.57, 93.1125) -> (302.57, 79.3129) projected
  line L143 (302.57, 79.3129) -> (288.771, 79.3129) projected
  line L144 (302.57, 79.3129) -> (288.771, 79.3129) projected
  line L145 (282.271, 88.4135) -> (283.096, 88.4135) projected
  line L146 (282.271, 88.4135) -> (283.096, 88.4135) projected
  line L147 (282.271, 91.6421) -> (282.271, 88.4135) projected
  line L148 (282.271, 91.6421) -> (282.271, 88.4135) projected
  line L149 (302.57, 93.1125) -> (302.57, 79.3129) projected
  line L150 (302.57, 93.1125) -> (302.57, 79.3129) projected
  line L151 (283.096, 88.4135) -> (283.096, 85.8132) projected
  line L152 (283.096, 88.4135) -> (283.096, 85.8132) projected
  line L153 (275.721, 91.6421) -> (282.271, 91.6421) projected
  line L154 (275.721, 91.6421) -> (282.271, 91.6421) projected
  line L155 (283.096, 85.8132) -> (282.271, 85.8132) projected
  line L156 (283.096, 85.8132) -> (282.271, 85.8132) projected
  line L157 (275.721, 88.4135) -> (275.721, 91.6421) projected
  line L158 (275.721, 88.4135) -> (275.721, 91.6421) projected
  line L159 (288.771, 79.3129) -> (288.771, 93.1125) projected
  line L160 (288.771, 79.3129) -> (288.771, 93.1125) projected
  line L161 (282.271, 85.8132) -> (282.271, 79.5433) projected
  line L162 (282.271, 85.8132) -> (282.271, 79.5433) projected
  line L163 (282.271, 79.5433) -> (280.545, 79.5433) projected
  line L164 (282.271, 79.5433) -> (280.545, 79.5433) projected
  line L165 (280.545, 79.5433) -> (280.545, 78.3428) projected
  line L166 (280.545, 79.5433) -> (280.545, 78.3428) projected
  line L167 (280.545, 78.3428) -> (277.446, 78.3428) projected
  line L168 (280.545, 78.3428) -> (277.446, 78.3428) projected
  line L169 (288.771, 93.1125) -> (302.57, 93.1125) projected
  line L170 (288.771, 93.1125) -> (302.57, 93.1125) projected
  line L171 (303.808, 119.826) -> (303.652, 119.844) projected
  line L172 (303.652, 119.844) -> (303.496, 119.849) projected
  line L173 (282.271, 91.6421) -> (282.271, 88.4135) projected
  line L174 (282.271, 85.8132) -> (282.271, 79.5433) projected
  line L175 (283.096, 85.8132) -> (282.271, 85.8132) projected
  line L176 (283.096, 85.8132) -> (282.271, 85.8132) projected
  line L177 (282.271, 88.4135) -> (283.096, 88.4135) projected
  line L178 (283.096, 88.4135) -> (283.096, 85.8132) projected
  line L179 (282.271, 88.4135) -> (283.096, 88.4135) projected
  line L180 (283.096, 88.4135) -> (283.096, 85.8132) projected
  line L181 (282.271, 91.6421) -> (282.271, 88.4135) projected
  line L182 (282.271, 85.8132) -> (282.271, 79.5433) projected
  line L183 (303.496, 0.1874) -> (303.652, 0.1929) projected
  line L184 (303.496, 0.1874) -> (303.652, 0.1929) projected
  line L185 (303.652, 0.1929) -> (303.808, 0.2122) projected
  line L186 (304.261, 0.339) -> (304.403, 0.4051) projected
  line L187 (304.261, 0.339) -> (304.403, 0.4051) projected
  line L188 (304.261, 0.339) -> (304.403, 0.4051) projected
  line L189 (304.115, 0.2853) -> (304.261, 0.339) projected
  line L190 (304.115, 0.2853) -> (304.261, 0.339) projected
  line L191 (304.115, 0.2853) -> (304.261, 0.339) projected
  line L192 (303.962, 0.2425) -> (304.115, 0.2853) projected
  line L193 (303.808, 0.2122) -> (303.962, 0.2425) projected
  line L194 (303.808, 0.2122) -> (303.962, 0.2425) projected
  line L195 (303.808, 0.2122) -> (303.962, 0.2425) projected
  line L196 (303.652, 0.1929) -> (303.808, 0.2122) projected
  line L197 (303.652, 0.1929) -> (303.808, 0.2122) projected
  line L198 (303.652, 0.1929) -> (303.808, 0.2122) projected
  line L199 (303.496, 0.1874) -> (303.652, 0.1929) projected
  line L200 (303.496, 0.1874) -> (303.652, 0.1929) projected
  line L201 (303.962, 0.2425) -> (304.115, 0.2853) projected
  line L202 (303.962, 0.2425) -> (304.115, 0.2853) projected
  line L203 (303.808, 0.2122) -> (303.962, 0.2425) projected
  line L204 (304.403, 0.4051) -> (304.541, 0.4823) projected
  line L205 (304.403, 0.4051) -> (304.541, 0.4823) projected
  line L206 (304.403, 0.4051) -> (304.541, 0.4823) projected
  line L207 (304.403, 0.4051) -> (304.541, 0.4823) projected
  line L208 (304.541, 0.4823) -> (304.672, 0.5691) projected
  line L209 (304.541, 0.4823) -> (304.672, 0.5691) projected
  line L210 (304.541, 0.4823) -> (304.672, 0.5691) projected
  line L211 (304.541, 0.4823) -> (304.672, 0.5691) projected
  line L212 (304.672, 0.5691) -> (304.794, 0.6656) projected
  line L213 (304.672, 0.5691) -> (304.794, 0.6656) projected
  line L214 (304.672, 0.5691) -> (304.794, 0.6656) projected
  line L215 (304.794, 0.6656) -> (304.91, 0.7731) projected
  line L216 (304.794, 0.6656) -> (304.91, 0.7731) projected
  line L217 (304.91, 0.7731) -> (305.016, 0.8875) projected
  line L218 (304.91, 0.7731) -> (305.016, 0.8875) projected
  line L219 (304.91, 0.7731) -> (305.016, 0.8875) projected
  line L220 (304.794, 0.6656) -> (304.91, 0.7731) projected
  line L221 (304.794, 0.6656) -> (304.91, 0.7731) projected
  line L222 (303.962, 0.2425) -> (304.115, 0.2853) projected
  line L223 (304.672, 0.5691) -> (304.794, 0.6656) projected
  line L224 (304.91, 0.7731) -> (305.016, 0.8875) projected
  line L225 (304.261, 0.339) -> (304.403, 0.4051) projected
  line L226 (305.201, 1.1424) -> (305.278, 1.2788) projected
  line L227 (251.92, 91.6421) -> (258.47, 91.6421) projected
  line L228 (251.92, 91.6421) -> (258.47, 91.6421) projected
  line L229 (251.92, 88.4135) -> (251.92, 91.6421) projected
  line L230 (251.92, 88.4135) -> (251.92, 91.6421) projected
  line L231 (251.095, 85.8132) -> (251.095, 88.4135) projected
  line L232 (251.095, 85.8132) -> (251.095, 88.4135) projected
  line L233 (251.92, 85.8132) -> (251.095, 85.8132) projected
  line L234 (251.92, 85.8132) -> (251.095, 85.8132) projected
  line L235 (251.095, 88.4135) -> (251.92, 88.4135) projected
  line L236 (251.095, 88.4135) -> (251.92, 88.4135) projected
  line L237 (251.92, 85.8132) -> (251.095, 85.8132) projected
  line L238 (251.095, 88.4135) -> (251.92, 88.4135) projected
  line L239 (251.92, 88.4135) -> (251.92, 91.6421) projected
  line L240 (251.92, 91.6421) -> (258.47, 91.6421) projected
  line L241 (258.47, 91.6421) -> (258.47, 88.4135) projected
  line L242 (258.47, 88.4135) -> (260.196, 88.4135) projected
  line L243 (258.47, 88.4135) -> (260.196, 88.4135) projected
  line L244 (251.92, 85.8132) -> (251.095, 85.8132) projected
  line L245 (273.995, 79.3129) -> (260.196, 79.3129) projected
  line L246 (273.995, 84.0133) -> (273.995, 79.3129) projected
  line L247 (273.995, 84.0133) -> (273.995, 79.3129) projected
  line L248 (275.721, 79.5433) -> (275.721, 84.0133) projected
  line L249 (275.721, 84.0133) -> (273.995, 84.0133) projected
  line L250 (275.721, 79.5433) -> (275.721, 84.0133) projected
  line L251 (275.721, 84.0133) -> (273.995, 84.0133) projected
  line L252 (273.995, 79.3129) -> (260.196, 79.3129) projected
  line L253 (273.995, 79.3129) -> (260.196, 79.3129) projected
  line L254 (273.995, 79.3129) -> (260.196, 79.3129) projected
  line L255 (260.196, 79.3129) -> (260.196, 84.0133) projected
  line L256 (260.196, 79.3129) -> (260.196, 84.0133) projected
  line L257 (273.995, 84.0133) -> (273.995, 79.3129) projected
  line L258 (273.995, 84.0133) -> (273.995, 79.3129) projected
  line L259 (260.196, 84.0133) -> (258.47, 84.0133) projected
  line L260 (260.196, 84.0133) -> (258.47, 84.0133) projected
  line L261 (258.47, 84.0133) -> (258.47, 79.5433) projected
  line L262 (275.721, 79.5433) -> (275.721, 84.0133) projected
  line L263 (275.721, 79.5433) -> (275.721, 84.0133) projected
  line L264 (275.721, 84.0133) -> (273.995, 84.0133) projected
  line L265 (275.721, 84.0133) -> (273.995, 84.0133) projected
  line L266 (273.995, 88.4135) -> (275.721, 88.4135) projected
  line L267 (273.995, 88.4135) -> (275.721, 88.4135) projected
  line L268 (273.995, 93.1125) -> (273.995, 88.4135) projected
  line L269 (273.995, 93.1125) -> (273.995, 88.4135) projected
  line L270 (260.196, 93.1125) -> (273.995, 93.1125) projected
  line L271 (260.196, 93.1125) -> (273.995, 93.1125) projected
  line L272 (258.47, 84.0133) -> (258.47, 79.5433) projected
  line L273 (256.745, 78.3428) -> (253.646, 78.3428) projected
  line L274 (256.745, 78.3428) -> (253.646, 78.3428) projected
  line L275 (253.646, 78.3428) -> (253.646, 79.5433) projected
  line L276 (260.196, 84.0133) -> (258.47, 84.0133) projected
  line L277 (260.196, 84.0133) -> (258.47, 84.0133) projected
  line L278 (258.47, 79.5433) -> (256.745, 79.5433) projected
  line L279 (258.47, 79.5433) -> (256.745, 79.5433) projected
  line L280 (258.47, 84.0133) -> (258.47, 79.5433) projected
  line L281 (258.47, 84.0133) -> (258.47, 79.5433) projected
  line L282 (260.196, 79.3129) -> (260.196, 84.0133) projected
  line L283 (260.196, 79.3129) -> (260.196, 84.0133) projected
  line L284 (253.646, 78.3428) -> (253.646, 79.5433) projected
  line L285 (253.646, 78.3428) -> (253.646, 79.5433) projected
  line L286 (253.646, 78.3428) -> (253.646, 79.5433) projected
  line L287 (256.745, 78.3428) -> (253.646, 78.3428) projected
  line L288 (256.745, 78.3428) -> (253.646, 78.3428) projected
  line L289 (253.646, 79.5433) -> (251.92, 79.5433) projected
  line L290 (253.646, 79.5433) -> (251.92, 79.5433) projected
  line L291 (253.646, 79.5433) -> (251.92, 79.5433) projected
  line L292 (253.646, 79.5433) -> (251.92, 79.5433) projected
  line L293 (258.47, 88.4135) -> (260.196, 88.4135) projected
  line L294 (258.47, 88.4135) -> (260.196, 88.4135) projected
  line L295 (260.196, 88.4135) -> (260.196, 93.1125) projected
  line L296 (260.196, 88.4135) -> (260.196, 93.1125) projected
  line L297 (258.47, 91.6421) -> (258.47, 88.4135) projected
  line L298 (258.47, 91.6421) -> (258.47, 88.4135) projected
  line L299 (251.92, 79.5433) -> (251.92, 85.8132) projected
  line L300 (251.92, 79.5433) -> (251.92, 85.8132) projected
  line L301 (251.92, 79.5433) -> (251.92, 85.8132) projected
  line L302 (251.92, 79.5433) -> (251.92, 85.8132) projected
  line L303 (241.146, 74.0625) -> (254.945, 74.0625) projected
  line L304 (241.146, 74.0625) -> (254.945, 74.0625) projected
  line L305 (231.621, 93.1125) -> (245.42, 93.1125) projected
  line L306 (231.621, 93.1125) -> (245.42, 93.1125) projected
  line L307 (231.621, 93.1125) -> (245.42, 93.1125) projected
  line L308 (241.146, 74.0625) -> (254.945, 74.0625) projected
  line L309 (241.146, 74.0625) -> (254.945, 74.0625) projected
  line L310 (245.42, 93.1125) -> (245.42, 79.3129) projected
  line L311 (245.42, 93.1125) -> (245.42, 79.3129) projected
  line L312 (245.42, 93.1125) -> (245.42, 79.3129) projected
  line L313 (245.42, 79.3129) -> (231.621, 79.3129) projected
  line L314 (245.42, 79.3129) -> (231.621, 79.3129) projected
  line L315 (245.42, 79.3129) -> (231.621, 79.3129) projected
  line L316 (231.621, 79.3129) -> (231.621, 93.1125) projected
  line L317 (231.621, 79.3129) -> (231.621, 93.1125) projected
  line L318 (231.621, 79.3129) -> (231.621, 93.1125) projected
  line L319 (245.42, 79.3129) -> (231.621, 79.3129) projected
  line L320 (231.621, 79.3129) -> (231.621, 93.1125) projected
  line L321 (231.621, 93.1125) -> (245.42, 93.1125) projected
  line L322 (222.096, 103.125) -> (222.096, 116.926) projected
  line L323 (235.895, 103.125) -> (222.096, 103.125) projected
  line L324 (235.895, 103.125) -> (222.096, 103.125) projected
  line L325 (245.42, 93.1125) -> (245.42, 79.3129) projected
  line L326 (226.37, 93.1125) -> (226.37, 79.3129) projected
  line L327 (258.47, 79.5433) -> (256.745, 79.5433) projected
  line L328 (258.47, 79.5433) -> (256.745, 79.5433) projected
  line L329 (277.446, 78.3428) -> (277.446, 79.5433) projected
  line L330 (277.446, 78.3428) -> (277.446, 79.5433) projected
  line L331 (256.745, 79.5433) -> (256.745, 78.3428) projected
  line L332 (256.745, 79.5433) -> (256.745, 78.3428) projected
  line L333 (256.745, 79.5433) -> (256.745, 78.3428) projected
  line L334 (256.745, 79.5433) -> (256.745, 78.3428) projected
  line L335 (254.945, 74.0625) -> (254.945, 60.2629) projected
  line L336 (254.945, 74.0625) -> (254.945, 60.2629) projected
  line L337 (254.945, 74.0625) -> (254.945, 60.2629) projected
  line L338 (254.945, 74.0625) -> (254.945, 60.2629) projected
  line L339 (264.958, 74.0625) -> (278.758, 74.0625) projected
  line L340 (264.958, 74.0625) -> (278.758, 74.0625) projected
  line L341 (264.958, 60.2629) -> (264.958, 74.0625) projected
  line L342 (264.958, 60.2629) -> (264.958, 74.0625) projected
  line L343 (278.758, 60.2629) -> (264.958, 60.2629) projected
  line L344 (278.758, 60.2629) -> (264.958, 60.2629) projected
  line L345 (278.758, 74.0625) -> (278.758, 60.2629) projected
  line L346 (278.758, 74.0625) -> (278.758, 60.2629) projected
  line L347 (277.446, 79.5433) -> (275.721, 79.5433) projected
  line L348 (277.446, 79.5433) -> (275.721, 79.5433) projected
  line L349 (254.945, 60.2629) -> (241.146, 60.2629) projected
  line L350 (254.945, 60.2629) -> (241.146, 60.2629) projected
  line L351 (226.37, 79.3129) -> (212.571, 79.3129) projected
  line L352 (278.758, 60.2629) -> (264.958, 60.2629) projected
  line L353 (257.813, 55.0125) -> (271.614, 55.0125) projected
  line L354 (257.813, 55.0125) -> (271.614, 55.0125) projected
  line L355 (264.958, 60.2629) -> (264.958, 74.0625) projected
  line L356 (264.958, 60.2629) -> (264.958, 74.0625) projected
  line L357 (278.758, 60.2629) -> (264.958, 60.2629) projected
  line L358 (264.958, 74.0625) -> (278.758, 74.0625) projected
  line L359 (264.958, 74.0625) -> (278.758, 74.0625) projected
  line L360 (278.758, 74.0625) -> (278.758, 60.2629) projected
  line L361 (278.758, 74.0625) -> (278.758, 60.2629) projected
  line L362 (302.57, 60.2629) -> (288.771, 60.2629) projected
  line L363 (302.57, 60.2629) -> (288.771, 60.2629) projected
  line L364 (288.771, 60.2629) -> (288.771, 74.0625) projected
  line L365 (288.771, 60.2629) -> (288.771, 74.0625) projected
  line L366 (288.771, 74.0625) -> (302.57, 74.0625) projected
  line L367 (288.771, 74.0625) -> (302.57, 74.0625) projected
  line L368 (302.57, 74.0625) -> (302.57, 60.2629) projected
  line L369 (302.57, 74.0625) -> (302.57, 60.2629) projected
  line L370 (302.57, 60.2629) -> (288.771, 60.2629) projected
  line L371 (302.57, 60.2629) -> (288.771, 60.2629) projected
  line L372 (288.771, 60.2629) -> (288.771, 74.0625) projected
  line L373 (288.771, 60.2629) -> (288.771, 74.0625) projected
  line L374 (302.57, 74.0625) -> (302.57, 60.2629) projected
  line L375 (302.57, 74.0625) -> (302.57, 60.2629) projected
  line L376 (288.771, 74.0625) -> (302.57, 74.0625) projected
  line L377 (288.771, 74.0625) -> (302.57, 74.0625) projected
  line L378 (302.57, 79.3129) -> (288.771, 79.3129) projected
  line L379 (302.57, 79.3129) -> (288.771, 79.3129) projected
  line L380 (305.496, 2.1869) -> (305.496, 117.85) projected
  line L381 (305.496, 2.1869) -> (305.496, 117.85) projected
  line L382 (283.52, 35.9625) -> (283.52, 22.163) projected
  line L383 (283.52, 35.9625) -> (283.52, 22.163) projected
  line L384 (288.771, 22.163) -> (288.771, 35.9625) projected
  line L385 (288.771, 22.163) -> (288.771, 35.9625) projected
  line L386 (302.57, 35.9625) -> (302.57, 22.163) projected
  line L387 (302.57, 35.9625) -> (302.57, 22.163) projected
  line L388 (305.496, 2.1869) -> (305.496, 117.85) projected
  line L389 (305.496, 2.187) -> (305.496, 117.85) projected
  line L390 (302.57, 22.163) -> (288.771, 22.163) projected
  line L391 (302.57, 22.163) -> (288.771, 22.163) projected
  line L392 (288.771, 16.9127) -> (302.57, 16.9127) projected
  line L393 (288.771, 16.9127) -> (302.57, 16.9127) projected
  line L394 (302.57, 16.9127) -> (302.57, 3.113) projected
  line L395 (302.57, 16.9127) -> (302.57, 3.113) projected
  line L396 (288.771, 3.113) -> (288.771, 16.9127) projected
  line L397 (288.771, 3.113) -> (288.771, 16.9127) projected
  line L398 (302.57, 3.113) -> (288.771, 3.113) projected
  line L399 (302.57, 3.113) -> (288.771, 3.113) projected
  line L400 (302.57, 41.2129) -> (288.771, 41.2129) projected
  line L401 (302.57, 41.2129) -> (288.771, 41.2129) projected
  line L402 (288.771, 41.2129) -> (288.771, 55.0125) projected
  line L403 (288.771, 41.2129) -> (288.771, 55.0125) projected
  line L404 (288.771, 55.0125) -> (302.57, 55.0125) projected
  line L405 (288.771, 55.0125) -> (302.57, 55.0125) projected
  line L406 (288.771, 35.9625) -> (302.57, 35.9625) projected
  line L407 (288.771, 35.9625) -> (302.57, 35.9625) projected
  line L408 (302.57, 55.0125) -> (302.57, 41.2129) projected
  line L409 (302.57, 55.0125) -> (302.57, 41.2129) projected
  line L410 (283.52, 22.163) -> (269.721, 22.163) projected
  line L411 (283.52, 22.163) -> (269.721, 22.163) projected
  line L412 (269.721, 22.163) -> (269.721, 35.9625) projected